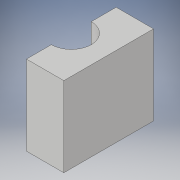
# Autodesk Inventor part: Lower Base Bearing Holder
Saved by Autodesk Inventor 2017 (Build 210142000, 142)
## iProperties
Created: 2018-10-30
Part Number: Lower Base Bearing Holder
Material: Generic
Document SubType Name: Modeling
Designer: 623516
Density: 1 g/cm^3
Appearance: Default
Author: 623516
Autodesk Inventor part; units mm, degrees
ref_plane "YZ Plane" through (0, 0, 0) normal (1, 0, 0) x (0, 1, 0)
ref_plane "XZ Plane" through (0, 0, 0) normal (0, 1, 0) x (-1, 0, 0)
ref_plane "XY Plane" through (0, 0, 0) normal (0, 0, 1) x (1, 0, 0)
sketch "Sketch1" plane through (0, 0, 0) normal (0, 1, 0) x (-1, 0, 0)
  line L0 (0, 0) -> (7.5, 0)
  line L1 (7.5, -18) -> (0, -18)
  line L2 (0, -18) -> (0, 0)
  arc A0 (7.5, -5) -> (7.5, -13) centre (7.5, -9) ccw
  line L3 (7.5, -18) -> (7.5, -13)
  line L4 (7.5, -5) -> (7.5, 0)
  dimension "d0" = 7.5
  dimension "d1" = 18
  dimension "d5" = 4
  dimension "d6" = 0
  dimension "d7" = 5
  dimension "d8" = 0
  constraints: 10 end point, 2 parallel, 2 point on circle, 1 centre point, 1 horizontal, 1 perpendicular, 1 vertical
  measures "d0" distance of L1.start L1.end
  measures "d1" distance of L0.end L1.start
  measures "d5" radius of A0
  measures "d6" distance between parallel lines of L4 L3
  measures "d7" distance from line of L4.start L0
  measures "d8" distance from line of A0.centre L4
extrude "Extrusion2" add sketch "Sketch1" along normal blind 16
body "Solid2"
